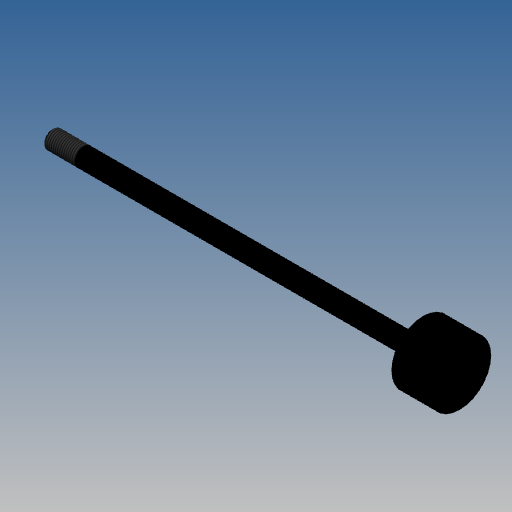
# Autodesk Inventor part: C-176-DP0000_rod
Saved by Autodesk Inventor 2020 (Build 240168000, 168)
## iProperties
Created: 2020-02-18
Part Number: C-176-DP0000_rod
Material: Generic
Catalog Web Link: www.cadenas.de
Description: Standard Air Cylinder_rod-Original Line - Standard Air Cylinders
Vendor: BIMBA
Document SubType Name: Modeling
Designer: psadmin
Manufacturer: BIMBA
Mass: 47.5128 g
Surface Area: 128.452 cm^2
Volume: 47.5128 cm^3
Density: 1 g/cm^3
Appearance: PSOLRGB-0-0-0
Category: PARTsolutions
Company: BIMBA
PSOL_IDENT_0: {$CADENAS_DATA\23d-libs\bimba\bimba_brand\bimba_imperial\bimba_full_line\original_line_cylinders\sta
PSOL_IDENT_1: ndard_air_cylinders\rod.prj},333 {VTYP=3D},{NB=C-176-DP0000_rod},{LINA=C-176-DP0000_rod},{NN=Standar
PSOL_IDENT_2: d Air Cylinder_rod},{DATE=10.02.2020 11:55:59},{GEOMDATE=27.08.2019 11:00:52},{VERSION=},{LINEID=80}
PSOL_IDENT_3: ,{WBVAR=STROKE,ACTING,MNT,DER,NR,BM,CO,M,EE,EEL,K,Q,Y,F,G,T,B,H,SER,SR,NT,W,E,HL,ST,STP,PRC,PB,COLOR
PSOL_IDENT_4: 1,FCD,RCD,BCD,ZHJ},{WBNUMERIC=STROKE,EEL,COLOR1,FCD,RCD,BCD,ZHJ}  {NB=C-176-DP0000_rod},{LINA=C-176-
PSOL_IDENT_5: DP0000_rod},{KT=DUMMY},{PN=C-176-DP000},{DASH=-},{BORE=1.50000000},{BOREPN=17},{STROKE=6.000},{STROK
PSOL_IDENT_6: EALG=[0.001:50/0.001]},{STROKE1=6.000},{ACTING=D},{ACTINGALG= '' , 'Single Acting' , 'R' , 'Reverse
PSOL_IDENT_7: Single Acting' , 'D' , 'Double Acting' },{ACTINGPN=D},{MNT=P},{MNTALG= '' , 'Front Nose Mounting' , '
PSOL_IDENT_8: P' , 'Rear Pivot Mounting' , 'X' , 'Universal Pivot Mounting or Double End Mounting' , 'BF' , 'Front
PSOL_IDENT_9: Block Mounting' , 'BR' , 'Rear Block Mounting for Vertical Positioning' , 'BFT' , 'Front Block Trun
PSOL_IDENT_10: nion Mounting' , 'BRT' , 'Rear Block Trunnion Mounting' },{TYPE=C-},{MNTPN=P},{DER=},{DERALG= '' , '
PSOL_IDENT_11: N/A' },{NR=},{NRALG= '' , 'N/A' },{NRPN=},{BM=},{BMALG= '' , 'N/A' },{BMPN=},{CO=},{COALG= '' , 'N/A'
PSOL_IDENT_12: },{M=},{MALG= '', 'Without Magnet', 'M', 'With Magnet' },{EE=},{EEL=0},{EEMAX=6},{EEALG= '', 'Witho
PSOL_IDENT_13: ut Extra Extension', 'EE', 'With Extra Extension' },{EELALG=0},{EEPN=},{EEPN1=0.000},{K=},{KALG= '',
PSOL_IDENT_14: 'Standard' , 'K' , 'Ports Rotated 90deg' },{KPN=},{Q=},{QALG= '' , 'Without Side Ported Rear Head'
PSOL_IDENT_15: , 'Q' , 'With Side Ported Rear Head' },{QPN=},{Y=},{YALG= '' , 'Without Pivot Bushing' , 'Y' , 'With
PSOL_IDENT_16: Pivot Bushing' },{YPN=},{F=},{FALG= '', 'Standard', 'F', 'Molycoated Body' },{FPN=},{G=},{GPN=},{T=
PSOL_IDENT_17: },{TALG= '' , 'Standard' , 'N' , 'Low Temperature' , 'V' , 'High Temperature' },{NPN=},{VPN=},{B=},{
PSOL_IDENT_18: BALG= '', 'Without Bumper' , 'B' , 'With Bumper' },{BPN=},{H=},{HALG= '', 'N/A' },{HPN=},{SER=},{SER
PSOL_IDENT_19: ALG= '' , 'Without Spring Extend/Return' , 'JS' , 'With Spring Return' , 'JR' , 'With Spring Extend'
PSOL_IDENT_20: },{SR=C},{SRALG= 'C' , 'Carbon Steel Rod' , 'SR' , '303 Stainless Steel Rod' , '' , '303 Stainless
PSOL_IDENT_21: Steel Rod1' },{SRPN=C},{SRCON=1},{NT=},{NTPN=},{W=},{WALG= '' , 'Without Wiper' , 'W' , 'With Wiper'
PSOL_IDENT_22: },{WPN=},{E=},{EALG= '' , 'Without Special Lube and Seals' , 'E' , 'With Special Lube and Seals' },
PSOL_IDENT_23: {EPN=},{HL=},{HLALG= '' , 'Wihout Low Pressure Hydraulic' , 'HL' , 'With Low Pressure Hydraulic' },{
PSOL_IDENT_24: ST=},{STALG= '' , 'Without Switch Track' , 'T' , 'With Switch Track' },{STP=},{STPALG= '' , 'N/A' },
PSOL_IDENT_25: {STPN=},{PRC=},{PRCALG= '' , 'Without Piston Rod Clevis' , 'D-166-1' , 'With Piston Rod Clevis' },{P
PSOL_IDENT_26: RCPN=},{PB=},{PBALG= '' , 'Without Pivot Bracket' , 'D-167' , 'With Pivot Bracket' },{PBPN=},{TLEN=7
PSOL_IDENT_27: .3025},{TEXT=0.5},{SPACE=0.285714},{FRAC=45.3800},{RGCON=},{RGDACCON=R},{RHCON=P},{RHCONON=1},{RHACC
PSOL_IDENT_28: ON=R},{FNUTCON=0},{RNUTCON=0},{FNUTPN=},{RNUTPN=},{FNUTTRANS=0.0000},{RNUTTRANS=0.0000},{VHOLECON=0}
PSOL_IDENT_29: ,{A1=1.8750},{A1N=1.3120},{A1P=1.8750},{A1B=2.3750},{A4=0.2525},{A4N=0.5000},{A4P=0.2525},{A5=0.0400
PSOL_IDENT_30: },{A1H=1.75},{A1NH=0.6880},{A1PH=1.7500},{A1BH=1.3750},{A1SH=1.5000},{A2H=0.2500},{A2NH=0.2500},{LEN
PSOL_IDENT_31: GTH=4.3800},{LENGTH1=4.3800},{LENGTH2=4.4400},{MUL=6.0000},{MUL11=6.0000},{MUL22=16.1400},{MUL33=10.
PSOL_IDENT_32: 1400},{MUL2=6.0000},{MUL211=6.0000},{MUL222=2.6900},{MUL233=1.6900},{SSS=12.0000},{RGLEN=1.6625},{RH
PSOL_IDENT_33: LEN=1.1650},{SSS1=7.0000},{A13=1.3750},{THDLEN1=0.7500},{THD1=0.4375},{TAB=UNF},{THDLEN=0.7500},{THD=
PSOL_IDENT_34: 0.4375},{OD=1.5115},{RODL=9.7550},{PL=0.8800},{RODDIA=0.4370},{HEX=0.4370},{RODTRANS=0.0000},{G1=0.0
PSOL_IDENT_35: 000},{ON=0},{G5=0.0000},{DERLEN=8.6250},{THOLE=0.2500},{WF=0.3800},{BADD=0.0000},{MADD=0.0000},{NVAD
PSOL_IDENT_36: D=0.000},{JRADD=0.00000},{COLOR=0.00,0.00,0.00,0.00},{GROOVE=1},{HOL=0},{D7=0.3775},{H1=1.6160},{D1=
PSOL_IDENT_37: 1.5565},{D1RH=1.5565},{D1P=1.5800},{D1B=1.5565},{D1N=1.5565},{D1NRH=1.5565},{D1BRH=1.5800},{D1PRH=1.
PSOL_IDENT_38: 5565},{BOZO=0},{HADD=0.000},{COLOR1=0},{DEFL=0.0000},{HEXL=0.0000},{SSADD=0.0000},{WFL=0.2500},{MOVE=
PSOL_IDENT_39: 0.2500},{PRCL2=0.75000},{PRCB=0.22000},{PRCTRANS=0.22000},{FCD=0},{RCD=0},{BCD=0},{ZHJ=0.000}
NN: Standard Air Cylinder_rod
NT: Standard
NB: C-176-DP0000_rod
NBSYN: $PN.$COLOR1._rod
LINA: C-176-DP0000_rod
PN: C-176-DP000
BORE: 1.5
BOREPN: 17
STROKE: 6
ACTING: Double Acting
MNT: Rear Pivot Mounting
DER: N/A
NR: N/A
BM: N/A
CO: N/A
M: Without Magnet
EE: Without Extra Extension
EEL: 0
K: Standard
Q: Without Side Ported Rear Head
Y: Without Pivot Bushing
F: Standard
G: Without Magnalube Lubrication
T: Standard
B: Without Bumper
H: N/A
SER: Without Spring Extend/Return
SR: Carbon Steel Rod
W: Without Wiper
E: Without Special Lube and Seals
HL: Wihout Low Pressure Hydraulic
ST: Without Switch Track
STP: N/A
PRC: Without Piston Rod Clevis
PB: Without Pivot Bracket
A1N: 1.312
A1P: 1.875
A1B: 2.375
A4N: 0.5
A4P: 0.2525
A5: 0.04
A1NH: 0.688
A1PH: 1.75
A1BH: 1.375
A1SH: 1.5
A2NH: 0.25
A13: 1.375
THDLEN1: 0.75
THD1: 0.4375
TAB: UNF
OD: 1.5115
RODDIA: 0.437
HEX: 0.437
G1: 0
G5: 0
THOLE: 0.25
WF: 0.38
GROOVE: 1
D7: 0.3775
D1P: 1.58
D1B: 1.5565
D1N: 1.5565
D1NRH: 1.5565
D1BRH: 1.58
D1PRH: 1.5565
COLOR1: 0
FCD: 0
RCD: 0
BCD: 0
ZHJ: 0
SUPPLIER: BIMBA
ARTICLENO: C-176-DP0000_rod
BOMINFO: C-176-DP0000_rod
CREATOR: CADENAS GmbH
Title: C-176-DP0000_rod
Author: Cadenas PARTsolutions
Comments: Original Line - Standard Air Cylinders
Autodesk Inventor part; units mm, degrees
sketch "Sketch_1" plane through (0, 0, 0) normal (0, 0, 1) x (1, 0, 0)
  line L0 (222.377, 0) -> (-6.35, 0)
  line L1 (-6.35, 0) -> (-6.35, 5.5499)
  line L2 (-6.35, 5.5499) -> (200.025, 5.5499)
  line L3 (200.025, 5.5499) -> (200.025, 19.1453)
  line L4 (200.025, 19.1453) -> (222.377, 19.1453)
  line L5 (222.377, 19.1453) -> (222.377, 0)
  line L6 (222.377, 0) -> (-6.35, 0)
  constraints: 14 end point
revolve "Revolution1" add sketch "Sketch_1" angle 360 about axis through (222.377, 0, 0) along (1, 0, 0)
sketch "Sketch_3" plane through (0, 0, 0) normal (0, 0, 1) x (1, 0, 0)
  line L0 (-6.35, 0) -> (-25.4, 0)
  line L1 (-25.4, 0) -> (-25.4, 4.8006)
  line L2 (-25.4, 4.8006) -> (-24.6443, 5.5563)
  line L3 (-24.6443, 5.5563) -> (-6.35, 5.5563)
  line L4 (-6.35, 5.5563) -> (-6.35, 0)
  line L5 (-6.35, 0) -> (-25.4, 0)
  constraints: 12 end point
revolve "Revolution2" add sketch "Sketch_3" angle 360 about axis through (-6.35, 0, 0) along (1, 0, 0)
thread "Thread1" size "7/16-20 UNF" class "2A" standard "ANSI Unified Screw Threads" full length
sketch "Sketch_10" plane through (-6.35, 0, 0) normal (1, 0, 0) x (0, 0, -1)
  line L0 (-11.0998, -11.0998) -> (11.0998, -11.0998)
  line L1 (11.0998, -11.0998) -> (11.0998, 11.0998)
  line L2 (11.0998, 11.0998) -> (-11.0998, 11.0998)
  line L3 (-11.0998, 11.0998) -> (-11.0998, -11.0998)
  line L4 (-4.826, -5.5499) -> (4.826, -5.5499)
  line L5 (4.826, -5.5499) -> (4.826, 5.5499)
  line L6 (4.826, 5.5499) -> (-4.826, 5.5499)
  line L7 (-4.826, 5.5499) -> (-4.826, -5.5499)
  constraints: 16 end point
extrude "Extrusion1" cut sketch "Sketch_10" along normal blind 6.35
ref_plane "dia1_XY" through (-6.35, 5.5499, 0) normal (1, 0, 0) x (0, 0, -1)
ref_plane "dia1_YZ" through (-6.35, 5.5499, 0) normal (0, 0, -1) x (0, 1, 0)
ref_plane "dia1_ZX" through (-6.35, 5.5499, 0) normal (0, 1, 0) x (1, 0, 0)
ref_plane "dia12_XY" through (0, 0, 19.7675) normal (1, 0, 0) x (0, 0, -1)
ref_plane "dia12_YZ" through (0, 0, 19.7675) normal (0, 0, -1) x (0, 1, 0)
ref_plane "dia12_ZX" through (0, 0, 19.7675) normal (0, 1, 0) x (1, 0, 0)
ref_plane "dia2_XY" through (-6.35, -5.5499, 0) normal (1, 0, 0) x (0, 0, -1)
ref_plane "dia2_YZ" through (-6.35, -5.5499, 0) normal (0, 0, -1) x (0, 1, 0)
ref_plane "dia2_ZX" through (-6.35, -5.5499, 0) normal (0, 1, 0) x (1, 0, 0)
ref_plane "dia22_XY" through (0, 0, -19.7675) normal (1, 0, 0) x (0, 0, -1)
ref_plane "dia22_YZ" through (0, 0, -19.7675) normal (0, 0, -1) x (0, 1, 0)
ref_plane "dia22_ZX" through (0, 0, -19.7675) normal (0, 1, 0) x (1, 0, 0)
ref_plane "rl1_XY" through (-25.4, 0, 0) normal (1, 0, 0) x (0, 0, -1)
ref_plane "rl1_YZ" through (-25.4, 0, 0) normal (0, 0, -1) x (0, 1, 0)
ref_plane "rl1_ZX" through (-25.4, 0, 0) normal (0, 1, 0) x (1, 0, 0)
ref_plane "rl2_XY" through (-6.35, 0, 0) normal (1, 0, 0) x (0, 0, -1)
ref_plane "rl2_YZ" through (-6.35, 0, 0) normal (0, 0, -1) x (0, 1, 0)
ref_plane "rl2_ZX" through (-6.35, 0, 0) normal (0, 1, 0) x (1, 0, 0)
ref_plane "rod_cp_XY" through (0, 0, 0) normal (1, 0, 0) x (0, 0, -1)
ref_plane "rod_cp_YZ" through (0, 0, 0) normal (0, 0, -1) x (0, 1, 0)
ref_plane "rod_cp_ZX" through (0, 0, 0) normal (0, 1, 0) x (1, 0, 0)
ref_plane "thd1_XY" through (-25.4, 5.5563, 0) normal (1, 0, 0) x (0, 0, -1)
ref_plane "thd1_YZ" through (-25.4, 5.5563, 0) normal (0, 0, -1) x (0, 1, 0)
ref_plane "thd1_ZX" through (-25.4, 5.5563, 0) normal (0, 1, 0) x (1, 0, 0)
ref_plane "thd2_XY" through (-25.4, -5.5563, 0) normal (1, 0, 0) x (0, 0, -1)
ref_plane "thd2_YZ" through (-25.4, -5.5563, 0) normal (0, 0, -1) x (0, 1, 0)
ref_plane "thd2_ZX" through (-25.4, -5.5563, 0) normal (0, 1, 0) x (1, 0, 0)
ref_plane "to_rod_clevis_XY" through (-30.988, 0, 0) normal (1, 0, 0) x (0, 0, -1)
ref_plane "to_rod_clevis_YZ" through (-30.988, 0, 0) normal (0, 0, -1) x (0, 1, 0)
ref_plane "to_rod_clevis_ZX" through (-30.988, 0, 0) normal (0, 1, 0) x (1, 0, 0)
ref_plane "wf1_XY" through (-6.35, 0, 0) normal (1, 0, 0) x (0, 0, -1)
ref_plane "wf1_YZ" through (-6.35, 0, 0) normal (0, 0, -1) x (0, 1, 0)
ref_plane "wf1_ZX" through (-6.35, 0, 0) normal (0, 1, 0) x (1, 0, 0)
ref_plane "wf2_XY" through (0, 0, 0) normal (1, 0, 0) x (0, 0, -1)
ref_plane "wf2_YZ" through (0, 0, 0) normal (0, 0, -1) x (0, 1, 0)
ref_plane "wf2_ZX" through (0, 0, 0) normal (0, 1, 0) x (1, 0, 0)
ref_plane "wfw1_XY" through (-6.35, 0, -4.826) normal (0, 1, 0) x (1, 0, 0)
ref_plane "wfw1_YZ" through (-6.35, 0, -4.826) normal (1, 0, 0) x (0, 0, -1)
ref_plane "wfw1_ZX" through (-6.35, 0, -4.826) normal (0, 0, -1) x (0, 1, 0)
ref_plane "wfw2_XY" through (-6.35, 0, 4.826) normal (0, 1, 0) x (1, 0, 0)
ref_plane "wfw2_YZ" through (-6.35, 0, 4.826) normal (1, 0, 0) x (0, 0, -1)
ref_plane "wfw2_ZX" through (-6.35, 0, 4.826) normal (0, 0, -1) x (0, 1, 0)
body "Solid1"
